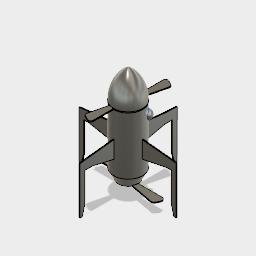
doro-nn (Autodesk Fusion 360 design; units mm, degrees)
Autodesk Fusion 360 part; units mm, degrees
sketch "スケッチ1" plane through (0, 0, 0) normal (0, 1, 0) x (1, 0, 0)
  circle A0 centre (0, 0) radius 30
extrude "押し出し1" add sketch "スケッチ1" along normal blind 120 makes body 1
sketch "スケッチ2" plane through (0, 120, 0) normal (0, 1, 0) x (-1, 0, 0)
  circle A0 centre (0, 0) radius 30
  line L0 (0, -30) -> (0, -71.9098)
  line L1 (-7.2361, -76.382) -> (-16.3784, -71.8108)
  line L2 (-19.0069, -66.1825) -> (-10, -28.2843)
  line L3 (-0.2283, 29.9991) -> (-0.2283, 72.024)
  line L4 (7.0078, 76.4961) -> (16.4276, 71.7862)
  line L5 (19.0471, 66.1212) -> (9.7717, 28.3639)
  arc A1 (19.0471, 66.1212) -> (16.4276, 71.7862) centre (14.1915, 67.3141) ccw
  arc A2 (7.0078, 76.4961) -> (-0.2283, 72.024) centre (4.7717, 72.024) ccw
  arc A3 (-7.2361, -76.382) -> (0, -71.9098) centre (-5, -71.9098) ccw
  arc A4 (-19.0069, -66.1825) -> (-16.3784, -71.8108) centre (-14.1424, -67.3386) ccw
  dimension "d4" = 10
  dimension "d5" = 10
  dimension "d6" = 5
  measures "d4" distance of L0.start L2.end
  measures "d5" distance of L3.start L5.end
  measures "d6" radius of A1
extrude "押し出し2" add sketch "スケッチ2" against normal blind 2 contours A0 L3 L4 L5 A1 A2 | A0 L0 L1 L2 A3 A4 bodies 1
sketch "スケッチ3" plane through (0, 0, 0) normal (0, 0, 1) x (1, 0, 0)
  arc A0 (0, 180) -> (-30, 120) centre (37.9269, 123.5366) ccw
  line L0 (0, 120) -> (-30, 120)
  line L1 (0, 180) -> (0, 120)
  line L2 (-30, 120) -> (0, 120)
  line L3 (30, 120) -> (0.2283, 120)
  point P0 (0, 120)
  point P1 (0, 120)
revolve "回転1" add sketch "スケッチ3" angle 360 about axis through (0, 180, 0) along (0, -1, 0) bodies 1
ref_plane "作業平面1" through (28.9945, 76.9354, 7.7019) normal (0.966483, 0, 0.25673) x (-0.25673, 0, 0.966483)
sketch "スケッチ6" plane through (0, 0, 0) normal (1, 0, 0) x (0, 0, -1)
ref_plane "作業平面2" through (-27.9593, 45.2213, -10.8756) normal (-0.931976, 0, -0.36252) x (0.36252, 0, -0.931976)
sketch "スケッチ7" plane through (-27.9593, 45.2213, -10.8756) normal (-0.931976, 0, -0.36252) x (0.36252, 0, -0.931976)
sketch "スケッチ8" plane through (0, 0, 0) normal (0, 0, 1) x (1, 0, 0)
  line L0 (30, 65) -> (80, 60)
  line L1 (30, 0) -> (-30, 0)
  line L2 (80, 60) -> (80, 40)
  line L3 (80, 40) -> (30, 30)
  line L4 (30, 30) -> (30, 65)
  line L5 (-30, 65) -> (-80, 60)
  line L6 (-80, 60) -> (-80, 40)
  line L7 (-80, 40) -> (-30, 30)
  line L8 (-30, 30) -> (-30, 65)
extrude "押し出し3" add sketch "スケッチ8" along normal mid plane 2 separate body makes body 2 at (46.6667, 45, 1) makes body 3 at (-46.6667, 45, 1)
ref_plane "作業平面3" through (-7.0418, 76.2541, -29.1618) normal (-0.234727, 0, -0.972061) x (0.972061, 0, -0.234727)
ref_plane "作業平面4" through (20.7952, 56.6758, -21.6231) normal (0.693173, 0, -0.720772) x (0.720772, 0, 0.693173)
sketch "スケッチ10" plane through (20.7952, 56.6758, -21.6231) normal (0.693173, 0, -0.720772) x (0.720772, 0, 0.693173)
  circle A0 centre (0, -40) radius 7.5
  dimension "d18" = 15
  measures "d18" diameter of A0
sphere "球プリミティブ2" add diameter 15 placed x (0.720772, 0, 0.693173) y (0, -1, 0) z (0.693173, 0, -0.720772) at (22.5955, 95.6487, -19.8918) bodies 1
sketch "スケッチ11" plane through (0, 0, 0) normal (1, 0, 0) x (0, 0, -1)
sketch "スケッチ12" plane through (0, 0, 0) normal (1, 0, 0) x (0, 0, -1)
  line L0 (-30, 65) -> (-75, 60)
  line L1 (-1, 65) -> (-1, 30)
  line L2 (-75, 60) -> (-75, 40)
  line L3 (-75, 40) -> (-30, 30)
  line L4 (-30, 30) -> (-30, 65)
  line L5 (30, 65) -> (75, 60)
  line L6 (75, 60) -> (75, 40)
  line L7 (75, 40) -> (30, 30)
  line L8 (30, 30) -> (30, 65)
extrude "押し出し4" add sketch "スケッチ12" along normal mid plane 2 separate body makes body 4 at (1, 45, -45) makes body 5 at (1, 45, 45)
sketch "スケッチ13" plane through (0, 120, 0) normal (0, 1, 0) x (-1, 0, 0)
  arc A0 (9.7717, 28.3639) -> (-0.2283, 29.9991) centre (0, 0) ccw
  line L0 (9.7717, 28.3639) -> (19.0471, 66.1212)
  arc A1 (19.0471, 66.1212) -> (16.4276, 71.7862) centre (14.1915, 67.3141) ccw
  line L1 (16.4276, 71.7862) -> (7.0078, 76.4961)
  arc A2 (7.0078, 76.4961) -> (-0.2283, 72.024) centre (4.7717, 72.024) ccw
  line L2 (-0.2283, 72.024) -> (-0.2283, 29.9991)
  circle A3 centre (0, 0) radius 30
  arc A4 (0, -30) -> (9.7717, 28.3639) centre (0, 0) ccw
  circle A5 centre (0, 0) radius 25
  line L3 (-10, -28.2843) -> (-8.3523, -23.5635)
  line L4 (8.1241, 23.6432) -> (9.7717, 28.3639)
  line L5 (0, -30) -> (-0.019, -25)
  line L6 (-0.2093, 24.9991) -> (-0.2283, 29.9991)
  line L7 (8.1241, 23.6432) -> (-0.2093, 24.9991)
  line L8 (-0.019, -25) -> (-8.3523, -23.5635)
  point P0 (-10, -28.2843)
extrude "押し出し5" cut sketch "スケッチ13" against normal blind 2 contours A3 A4 A5 L4 L5 | A3 A5 L3 L6 bodies 1
sketch "スケッチ14" plane through (0, 0, 0) normal (0, 0, 1) x (1, 0, 0)
  line L0 (30, 0) -> (-30, 0)
  line L1 (30, 0) -> (20, -20)
  line L2 (20, -20) -> (0, -20)
  line L3 (30, 0) -> (0, 0)
  line L4 (0, 0) -> (0, -20)
revolve "回転2" add sketch "スケッチ14" angle 360 about axis through (0, 0, 0) along (0, -1, 0) bodies 1
sketch "スケッチ15" plane through (0, -20, 0) normal (0, -1, 0) x (1, 0, 0)
  circle A0 centre (0, 0) radius 20
  line L0 (30, -1) -> (80, -1)
  line L1 (20, 0) -> (70.2918, 0)
  line L2 (75.6584, 8.6833) -> (72.0287, 15.9425)
  line L3 (65.5432, 19.154) -> (17.3205, 10)
  line L4 (-80, -1) -> (-30, -1)
  line L5 (-19.9985, -0.2448) -> (-70.2379, -0.2448)
  line L6 (-75.5912, -8.9545) -> (-72.033, -15.9838)
  line L7 (-65.5754, -19.1715) -> (-17.2493, -10.1224)
  arc A1 (-70.2379, -0.2448) -> (-75.5912, -8.9545) centre (-70.2379, -6.2448) ccw
  arc A2 (-72.033, -15.9838) -> (-65.5754, -19.1715) centre (-66.6798, -13.274) ccw
  arc A3 (72.0287, 15.9425) -> (65.5432, 19.154) centre (66.6622, 13.2592) ccw
  arc A4 (70.2918, 0) -> (75.6584, 8.6833) centre (70.2918, 6) ccw
  point P0 (20, 0)
  dimension "d25" = 6
  measures "d25" radius of A1
extrude "押し出し6" add sketch "スケッチ15" against normal blind 2 contours A0 L1 L2 L3 A3 A4 | A0 L5 L6 L7 A1 A2 bodies 1
sketch "スケッチ16" plane through (1, 0, 0) normal (1, 0, 0) x (0, 0, -1)
  line L0 (-30, 30) -> (-30, 65)
  line L1 (-30, 65) -> (-75, 60)
  line L2 (-75, 60) -> (-75, 40)
  line L3 (-75, 40) -> (-30, 30)
  line L4 (-75, 60) -> (-100.283, 57.1908)
  line L5 (-100.283, 57.1908) -> (-100.283, 40)
  line L6 (-100.283, 40) -> (-75, 40)
  line L7 (75, 60) -> (100.3261, 58.5954)
  line L8 (100.3261, 58.5954) -> (100.3261, 40)
  line L9 (100.3261, 40) -> (75, 40)
  line L10 (75, 60) -> (75, 40)
  line L11 (-90, 40) -> (-90, -40)
  line L12 (-90, -40) -> (-100.283, -40)
  line L13 (-100.283, -40) -> (-100.283, 40)
  line L14 (90, 40) -> (90, -40)
  line L15 (90, -40) -> (100, -40)
  line L16 (100, -40) -> (100.3261, 40)
  line L17 (-95.1415, -40) -> (-90, -20)
  line L18 (95, -40) -> (90, -20)
  point P0 (75, 60)
  point P1 (75, 40)
extrude "押し出し7" add sketch "スケッチ16" against normal blind 2 contours L2 L4 L5 L6 | L6 L11 L12 L13 L17 | L7 L8 L9 L10 | L9 L14 L15 L16 L18 bodies 4 5
sketch "スケッチ17" plane through (0, 0, 1) normal (0, 0, 1) x (1, 0, 0)
  line L0 (30, 30) -> (80, 40)
  line L1 (80, 40) -> (80, 60)
  line L2 (80, 60) -> (30, 65)
  line L3 (30, 65) -> (30, 30)
  line L4 (80, 60) -> (99.9007, 58.0099)
  line L5 (99.9007, 58.0099) -> (99.9007, 40)
  line L6 (99.9007, 40) -> (80, 40)
  line L7 (99.9007, 40) -> (99.9007, -40)
  line L8 (99.9007, -40) -> (95, -40)
  line L9 (95, -40) -> (89.9504, -40)
  line L10 (89.9504, -40) -> (89.9504, 40)
  line L11 (95, -40) -> (89.9504, -20.4108)
  dimension "d32" = 20
  measures "d32" distance of L1.end L4.end
sketch "スケッチ19" plane through (0, 0, 1) normal (0, 0, 1) x (1, 0, 0)
  line L0 (-30, 30) -> (-30, 65)
  line L1 (-30, 65) -> (-80, 60)
  line L2 (-80, 60) -> (-80, 40)
  line L3 (-80, 40) -> (-30, 30)
  line L4 (-80, 60) -> (-100.3708, 57.6959)
  line L5 (-100.3708, 57.6959) -> (-100.3708, 40)
  line L6 (-100.3708, 40) -> (-80, 40)
  line L7 (-90.1854, 40) -> (-90.1854, -40)
  line L8 (-90.1854, -40) -> (-100.3708, -40)
  line L9 (-100.3708, -40) -> (-100.3708, 40)
  line L10 (-95.2781, -40) -> (-90.1854, -19.8729)
extrude "押し出し8" add sketch "スケッチ19" against normal blind 2 contours L2 L4 L5 L6 | L6 L7 L8 L9 L10 bodies 3
extrude "押し出し9" add sketch "スケッチ17" against normal blind 2 contours L1 L4 L5 L6 | L6 L7 L8 L10 L11 bodies 2
sketch "スケッチ18" plane through (1, 0, 0) normal (1, 0, 0) x (0, 0, -1)
  line L0 (-30, 30) -> (-30, 65)
  line L1 (-30, 65) -> (-100.283, 57.1908)
  line L2 (-100.283, 57.1908) -> (-100.283, -40)
  line L3 (-100.283, -40) -> (-95.1415, -40)
  line L4 (-95.1415, -40) -> (-90, -20)
  line L5 (-90, -20) -> (-90, 40)
  line L6 (-90, 40) -> (-75, 40)
  line L7 (-75, 40) -> (-30, 30)
